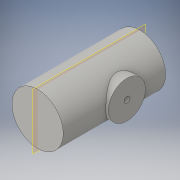
# Autodesk Inventor part: Camera
Saved by Autodesk Inventor 2016 (Build 200138000, 138)
## iProperties
Created: 2017-10-12
Part Number: Camera
Material: Generic
Document SubType Name: Modeling
Designer: Student
Density: 1 g/cm^3
Appearance: Default
Author: Student
Autodesk Inventor part; units mm, degrees
ref_plane "XZ Plane" through (0, 0, 0) normal (0, 1, 0) x (-1, 0, 0)
ref_plane "XY Plane" through (0, 0, 0) normal (0, 0, 1) x (1, 0, 0)
sketch "Sketch1" plane through (0, 0, 0) normal (0, 0, 1) x (1, 0, 0)
  circle A0 centre (0, 0) radius 13.5255
  dimension "d0" = 27.051
  constraints: 1 centre point, 1 coincident
  measures "d0" diameter of A0
extrude "Extrusion1" add sketch "Sketch1" along normal blind 54.0766
sketch "Sketch2" plane through (0, 0, 0) normal (1, 0, 0) x (0, 1, 0)
  circle A0 centre (0, 21.742) radius 9.8044
  point P0 (0, 0)
  dimension "d3" = 19.6088
  constraints: 1 centre point
  measures "d3" diameter of A0
extrude "Extrusion2" add sketch "Sketch2" along normal blind 14.8082
sketch "Sketch3" plane through (14.8082, 0, 21.742) normal (1, 0, 0) x (0, 0, -1)
  circle A0 centre (0, 0) radius 1.5
  point P0 (21.742, 0)
  dimension "d6" = 3
  constraints: 1 centre point
  measures "d6" diameter of A0
extrude "Extrusion3" cut sketch "Sketch3" against normal blind 14.8082
body "Solid1"
